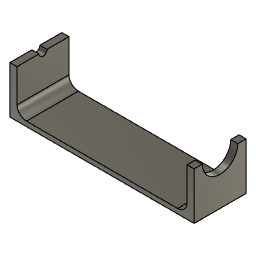
Simple Soilnoid Mount (Autodesk Fusion 360 design; units mm, degrees)
Autodesk Fusion 360 part; units mm, degrees
sketch "Sketch1" plane through (0, 0, 0) normal (0, 0, 1) x (1, 0, 0)
  line L0 (0, 0) -> (-78, 0)
  line L1 (-78, 0) -> (-78, 22)
  line L2 (-78, 22) -> (0, 22)
  line L3 (0, 22) -> (0, 0)
  dimension "d1" = 78
  dimension "d2" = 22
  constraint horizontal L0
  constraint vertical L1
  constraint horizontal L2
  constraint vertical L3
  constraint coincident L0.start L3.end
  measures "d1" distance of L0.start L0.end
  measures "d2" distance of L0.start L2.end
extrude "Extrude1" add sketch "Sketch1" along normal blind 2
sketch "Sketch2" plane through (0, 0, 0) normal (1, 0, 0) x (0, 1, 0)
  line L0 (0, 0) -> (22, 0)
  line L1 (22, 0) -> (22, 2)
  line L2 (22, 2) -> (0, 2)
  line L3 (0, 2) -> (0, 0)
  line L4 (0, 2) -> (0, 20)
  line L5 (0, 20) -> (22, 20)
  line L6 (22, 20) -> (22, 2)
  circle A0 centre (11, 20) radius 7.5
  dimension "d8" = 18
  dimension "d9" = 15
  constraint horizontal L0
  constraint vertical L1
  constraint horizontal L2
  constraint vertical L3
  constraint coincident L0.start L3.end
  constraint perpendicular L2 L4
  constraint perpendicular L4 L5
  constraint perpendicular L2 L6
  constraint midpoint L5 A0.centre
  measures "d8" distance of L2.end L4.end
  measures "d9" diameter of A0
extrude "Extrude2" add sketch "Sketch2" against normal blind 3 contours L2 L4 L5 L6 A0
sketch "Sketch3" plane through (-78, 0, 0) normal (-1, 0, 0) x (0, -1, 0)
  line L0 (-22, 0) -> (0, 0)
  line L1 (0, 0) -> (0, 2)
  line L2 (0, 2) -> (-22, 2)
  line L3 (-22, 2) -> (-22, 0)
  line L4 (0, 0) -> (-22, 0)
  line L5 (-22, 0) -> (-22, 2)
  line L6 (-22, 2) -> (0, 2)
  line L7 (0, 2) -> (0, 0)
  line L8 (0, 2) -> (0, 20)
  line L9 (0, 20) -> (-22, 20)
  line L10 (-22, 20) -> (-22, 2)
  circle A0 centre (-11, 20) radius 1.7
  dimension "d12" = 3.4
  constraint horizontal L4
  constraint vertical L5
  constraint horizontal L6
  constraint vertical L7
  constraint coincident L2.end L3.start
  constraint coincident L0.end L1.start
  constraint coincident L1.end L2.start
  constraint perpendicular L6 L8
  constraint perpendicular L7 L9
  constraint midpoint L9 A0.centre
  measures "d12" diameter of A0
extrude "Extrude3" add sketch "Sketch3" against normal blind 3 contours L2 L6 L8 L9 L10 A0
fillet "Fillet1" radius 4 2 edges at (-75, 11, 2) (-3, 11, 2)
equation "d1 = 81 mm - 3 mm"
